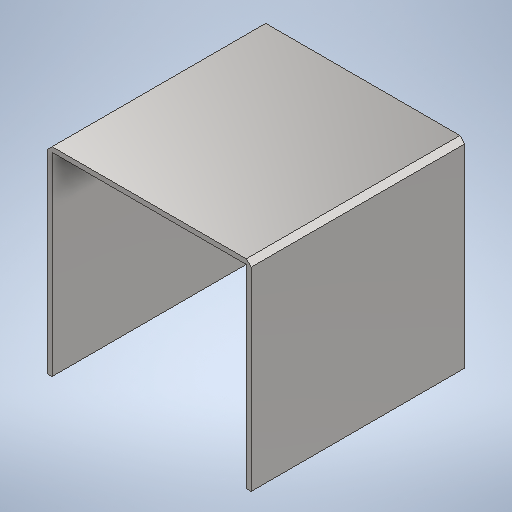
# Autodesk Inventor part: cover
Saved by Autodesk Inventor 2025 (Build 290162000, 162)
## iProperties
Created: 2024-10-02
Part Number: cover
Material: Generic
Document SubType Name: Modeling
Designer: DMIADX
Density: 1 g/cm^3
Appearance: Stainless - Brushed
Author: DMIADX
Autodesk Inventor part; units mm, degrees
ref_plane "YZ Plane" through (0, 0, 0) normal (1, 0, 0) x (0, 1, 0)
ref_plane "XZ Plane" through (0, 0, 0) normal (0, 1, 0) x (-1, 0, 0)
ref_plane "XY Plane" through (0, 0, 0) normal (0, 0, 1) x (1, 0, 0)
sketch "Sketch1" plane through (0, 0, 0) normal (0, 0, 1) x (1, 0, 0)
  line L0 (10, -10) -> (-10, -10)
  line L1 (-10, -10) -> (-10, 10)
  line L2 (-10, 10) -> (10, 10)
  line L3 (10, 10) -> (10, -10)
  line L4 (10, -10) -> (-10, 10) construction
  line L5 (-10, -10) -> (10, 10) construction
  line L6 (10.5, 10.5) -> (-10.5, 10.5)
  line L7 (-10.5, 10.5) -> (-10.5, -10.5)
  line L8 (-10.5, -10.5) -> (10.5, -10.5)
  line L9 (10.5, -10.5) -> (10.5, 10.5)
  line L10 (-10.5, -10) -> (10.5, -10)
  point P0 (0, 0)
  dimension "d0" = 20
  dimension "d1" = 20
  dimension "d2" = 0.5
  constraints: 22 end point, 4 parallel, 4 point on line, 2 midpoint, 2 perpendicular, 1 horizontal, 3 other
  measures "d0" distance of L1.end L2.end
  measures "d1" distance of L0.end L1.end
  measures "d2" distance between parallel lines of L2 L6
extrude "Extrusion1" add sketch "Sketch1" along normal mid plane 22 contours L3 L2 L1 L10 L7 L6 L9
chamfer "Chamfer1" distance 0.5 angle 45 2 edges at (10.5, 10.5, 0) (-10.5, 10.5, 0)
body "Solid1"
